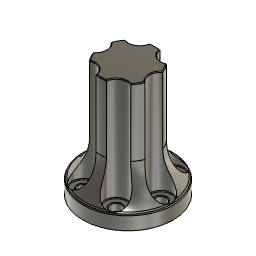
Motor_Shaft v4 (Autodesk Fusion 360 archive; units mm, degrees)
design "Motor_Shaft v4" references "Spring Washer BS 4464 - M4 - Type B Steel 100 HV Plain", "Forged Hexagon Socket Head Cap Screw ANSI B18.3.1M - M4x0.7 x 12 Steel Grade 8 Plain"
Autodesk Fusion 360 part; units mm, degrees
sketch "Sketch1" plane through (0, 0, 0) normal (0, 0, 1) x (1, 0, 0)
  circle A0 centre (0, 0) radius 16.5
  dimension "d1" = 33
  constraint coincident A0.centre origin
  measures "d1" diameter of A0
extrude "Extrude1" add sketch "Sketch1" along normal blind 5
sketch "Sketch2" plane through (0, 0, 5) normal (0, 0, 1) x (-1, 0, 0)
  circle A0 centre (0, 0) radius 16.5
  circle A1 centre (0, 0) radius 12 construction
  circle A2 centre (12, 0) radius 2.075
  circle A3 centre (6, 10.3923) radius 2.075
  circle A4 centre (-6, 10.3923) radius 2.075
  circle A5 centre (-12, 0) radius 2.075
  circle A6 centre (-6, -10.3923) radius 2.075
  circle A7 centre (6, -10.3923) radius 2.075
  circle A8 centre (0, 0) radius 10
  circle A9 centre (12, 0) radius 4.125
  circle A10 centre (6, 10.3923) radius 4.125
  circle A11 centre (-6, 10.3923) radius 4.125
  circle A12 centre (-12, 0) radius 4.125
  circle A13 centre (-6, -10.3923) radius 4.125
  circle A14 centre (6, -10.3923) radius 4.125
  dimension "d4" = 24
  dimension "d5" = 4.15
  dimension "d7" = 360
  dimension "d10" = 20
  dimension "d15" = 8.25
  dimension "d17" = 360
  constraint coincident A0.centre A1.centre
  constraint coincident A1 A2.centre
  constraint concentric A1 A8
  constraint concentric A2 A9
  measures "d4" diameter of A1
  measures "d5" diameter of A2
  measures "d10" diameter of A8
  measures "d15" diameter of A9
extrude "Extrude2" cut sketch "Sketch2" against normal blind 5.5 contours A2 A8 | A2 A8 | A3 A8 | A3 A8 | A7 A8 | A7 A8 | A4 A8 | A4 A8 | A6 A8 | A6 A8 | A5 A8 | A5 A8
extrude "Extrude3" add sketch "Sketch2" along normal blind 37 contours A2 A8 | A2 A8 A9 | A8 A9 A10 A11 A12 A13 A14 | A3 A8 A10 | A7 A8 A14 | A3 A8 | A7 A8 | A4 A8 A11 | A6 A8 A13 | A4 A8 | A6 A8 | A5 A8 A12 | A5 A8 picked at (9.9547, 0.1408) picked at (9.3357, 1.1161) picked at (3.7013, 8.643) picked at (3.7013, -8.643) picked at (4.987, 8.6378) picked at (4.987, -8.6378) picked at (-3.7013, 8.643) picked at (-3.7013, -8.643) picked at (-4.987, 8.6378) picked at (-4.987, -8.6378) picked at (-9.2988, 0.9985) picked at (-9.9741, 0)
sketch "Sketch3" plane through (0, 0, 0) normal (0, 1, 0) x (1, 0, 0)
  line L0 (-10, -5) -> (-16.5, -5)
  line L1 (-10, -5) -> (-10, -10)
  line L2 (-10, -10) -> (-16.5, -5)
  arc A0 (-10, -10) -> (-16.5, -5) centre (-15.1731, -10) ccw
  point P0 (-16.5, -5)
  point P1 (-9.9873, -5)
  point P2 (-9.9873, -5)
  dimension "d13" = 5
  constraint coincident P0 L0.end
  constraint perpendicular L0 L1
  constraint tangent L1 A0
  measures "d13" distance of L0.start L1.end
revolve "Revolve1" add sketch "Sketch3" angle 360 about axis through (0, 0, 1.75) along (0, 0, 1) contours L0 L1 A0 | L0 L2 A0
extrude "Extrude4" cut sketch "Sketch2" along normal blind 37 and the other way blind 1 contours A2 A8 | A2 A8 A9 | A2 A8 | A2 A8 A9 | A3 A8 A10 | A3 A8 A10 | A7 A8 A14 | A7 A8 A14 | A3 A8 | A3 A8 | A7 A8 | A7 A8 | A4 A8 A11 | A4 A8 A11 | A6 A8 A13 | A6 A8 A13 | A4 A8 | A4 A8 | A6 A8 | A6 A8 | A5 A8 A12 | A5 A8 A12 | A5 A8 | A5 A8
fillet "Fillet1" radius 15 6 edges at (0, -10, 10) (8.6603, -5, 10) (8.6603, 5, 10) (-8.6603, -5, 10) (-8.6603, 5, 10) (0, 10, 10)
sketch "Sketch4" plane through (0, 0, 0) normal (0, 0, -1) x (1, 0, 0)
  circle A0 centre (0, 0) radius 16.5
  circle A1 centre (0, 0) radius 15.25
  circle A2 centre (12, 0) radius 2.075
  circle A3 centre (-12, 0) radius 2.075
  circle A4 centre (6, 10.3923) radius 2.075
  circle A5 centre (6, -10.3923) radius 2.075
  circle A6 centre (-6, -10.3923) radius 2.075
  circle A7 centre (-6, 10.3923) radius 2.075
  dimension "d25" = 30.5
  constraint coincident A0.centre A1.centre
  measures "d25" diameter of A1
extrude "Extrude5" cut sketch "Sketch4" against normal blind 1 contours A1 | A2 | A3 | A4 | A5 | A6 | A7
chamfer "Chamfer1" distance 0.25 angle 45 1 faces at (-1.4005, 2.3241, 42)
chamfer "Chamfer1" distance 0.25 angle 45 6 faces at (3.9353, 10.5989, 3) (9.9353, 0.2066, 3) (-8.0647, 10.5989, 3) (-14.0647, 0.2066, 3) (3.9353, -10.1857, 3) (-8.0647, -10.1857, 3)
fillet "Fillet2" radius 0.25 1 edges at (-14.218, -5.5146, 1)
fillet "Fillet2" radius 0.5 1 edges at (-15.3834, -5.9667, 5)
fillet "Fillet2" radius 0.25 6 edges at (-2.1541, -11.884, 4) (9.8459, -11.884, 4) (-8.1541, -1.4917, 4) (-2.1541, 8.9006, 4) (9.8459, 8.9006, 4) (15.8459, -1.4917, 4)
thread "Thread1" [rolled back] thread offset 0 thread length 10
other "Washer7"
other "Washer8"
other "Washer9"
other "Washer10"
other "Washer11"
other "Washer12"
other "Screw13"
other "Screw14"
other "Screw15"
other "Screw16"
other "Screw17"
other "Screw18"

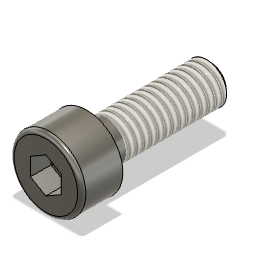
design "Forged Hexagon Socket Head Cap Screw ANSI B18.3.1M - M4x0.7 x 12 Steel Grade 8 Plain"
description: Forged Hexagon Socket Head Cap Screw ANSI B18.3.1M - M4x0.7 x 12
Autodesk Fusion 360 part; units mm, degrees
sketch "Sketch1" plane through (0, 0, 0) normal (0, 1, 0) x (1, 0, 0)
  line L0 (-2, 0) -> (-2, 12)
  line L1 (-2, 12) -> (0, 12)
  line L2 (0, 12) -> (0, -4)
  line L3 (-2, 0) -> (-3.5, 0)
  line L4 (-3.5, 0) -> (-3.5, -4)
  line L5 (-3.5, -4) -> (0, -4)
  dimension "d9" = 4
  dimension "d66" = 7
  dimension "d68" = 12
  dimension "d79" = 4
  constraint perpendicular L0 L1
  constraint collinear origin L1.end L2.end
  constraint perpendicular L0 L3
  constraint coincident origin L3
  constraint vertical L0
  constraint vertical L2
  constraint parallel L2 L4
  constraint coincident L2 L5.end
  constraint perpendicular L2 L5
  measures "d68" distance of origin L1.end
  measures "d79" distance of L3.end L4.end
revolve "Revolve1" add sketch "Sketch1" angle 360 about axis through (0, 0, -12) along (0, 0, 1)
ref_plane "WorkPlane1" through (0, 0, 4) normal (0, 0, 1) x (1, 0, 0)
sketch "Sketch6" plane through (0, 0, 4) normal (0, 0, 1) x (1, 0, 0)
  line L0 (-1.5, 0) -> (1.5, 0) construction
  line L1 (0, 0) -> (-1.5, 0.866)
  line L2 (-1.5, -0.866) -> (-1.5, 0.866)
  line L3 (-1.5, -0.866) -> (0, 0)
  dimension "d72" = 3
  dimension "d100" = 150
  constraint horizontal L0
  constraint midpoint L1.start L0
  constraint coincident L1.start L3.end
  constraint perpendicular L0 L2
  constraint midpoint L0.start L2
  constraint coincident L1.end L2.end
  measures "d72" distance of L0.start L0.end
  measures "d100" angle of L0 L1
extrude "Extrude1" cut sketch "Sketch6" against normal blind 2
pattern_circular "C-Pattern1" count 6 over 360 about axis through (0, 0, 1.75) along (0, 0, 1) of "Extrude1"
extrude "Extrude2" cut 1 faces at (0, -0.5774, 2) along direction (0, 0, -1) blind 2 draft -85
thread "Thread2" "ANSI Metric M Profile 4.0 M4x0.7 4g6g" major diameter 3.908 minor diameter 3.128 pitch 0.7 angle 60 resizes the face on face at (-1.9975, 0.0997, -8) from (0, 0, -1.8294) to (0, 0, -12)
fillet "Fillet4" radius 0.4 1 edges at (-3.2631, 1.2657, 4)
sketch "Sketch7" plane through (0, 0, 0) normal (0, 1, 0) x (1, 0, 0)
  line L0 (-2.04, 12) -> (-2.04, 11.5706)
  line L1 (-2.04, 11.5706) -> (-1.5706, 12)
  line L2 (0, 12) -> (0, -4)
  line L3 (-2.04, 12) -> (0, 12)
  dimension "d92" = 0.4294
  dimension "d98" = 1.5706
  dimension "d99" = 2.04
  constraint coincident L2.start L3.end
  constraint perpendicular L2 L3
  constraint coincident L1.end L3
  constraint perpendicular L0 L3
  measures "d92" vertical distance of L0.end L1.end
  measures "d98" horizontal distance of origin L1.end
  measures "d99" distance of origin L0
revolve "Revolve3" cut sketch "Sketch7" angle 360 about axis through (0, 0, 1.75) along (0, 0, 1)
equation "d9 = adsk_nomdia"
equation "adsk_nomlen = 12.00 mm"
equation "adsk_headh = 4.00 mm"
equation "adsk_headdia = 7.00 mm"
equation "adsk_nomdia = 4.00 mm"
equation "adsk_philwidth = 3.00 mm"
equation "d31 = -adsk_phildepth"
equation "adsk_phildepth = 2.00 mm"
equation "d66 = adsk_headdia"
equation "d68 = adsk_nomlen"
equation "d71 = adsk_headh"
equation "d72 = adsk_philwidth"
equation "d76 = -adsk_phildepth"
equation "d79 = adsk_headh"
equation "adsk_thrlen = 10.170585 mm"
equation "d84 = adsk_thrlen"
equation "d86 = adsk_nomdia * 0.1"
equation "d92 = adsk_startlen"
equation "adsk_startlen = 0.429415 mm"
equation "adsk_endpointdia = 3.14117 mm"
equation "d98 = adsk_endpointdia / 2"
equation "d99 = adsk_nomdia * 0.51"

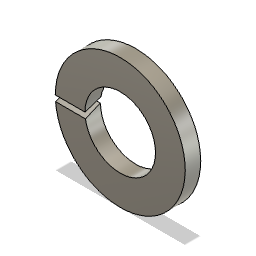
design "Spring Washer BS 4464 - M4 - Type B Steel 100 HV Plain"
description: Spring Washer BS 4464 - M4 - Type B
Autodesk Fusion 360 part; units mm, degrees
sketch "Sketch1" plane through (0, 0, 0) normal (0, 0, 1) x (1, 0, 0)
  circle A0 centre (0, 0) radius 3.775
  circle A1 centre (0, 0) radius 2.05
  dimension "d4" = 7.55
  dimension "d5" = 4.1
  constraint coincident A0.centre A1.centre
  measures "d4" diameter of A0
  measures "d5" diameter of A1
extrude "Extrude1" add sketch "Sketch1" along normal blind 0.9
ref_plane "WorkPlane1" through (12.125, 0, 0) normal (0, -0.34202, 0.939693) x (1, 0, 0)
ref_plane "WorkPlane2" through (12.125, -0.1539, 0.4229) normal (0, -0.34202, 0.939693) x (1, 0, 0)
sketch "Sketch2" plane through (12.125, -0.1539, 0.4229) normal (0, -0.34202, 0.939693) x (1, 0, 0)
  ellipse E0 centre (-12.125, 0.3078) end of major axis (-8.35, 0.3078) minor radius 3.5473
  ellipse E1 centre (-12.125, 0) end of major axis (-8.35, 0) minor radius 3.5473
  line L0 (-12.125, 0.3078) -> (-12.125, 0)
  line L1 (-12.125, 0.3078) -> (-16.051, 0.3078)
  line L2 (-12.125, 0) -> (-16.051, 0)
  line L3 (-16.051, 0) -> (-16.051, 0.3078)
  dimension "d15" = 3.926
  constraint coincident E0.centre L0.start
  constraint coincident E1.centre L0.end
  constraint perpendicular L0 L1
  constraint perpendicular L0 L2
  constraint vertical L3
  measures "d15" distance of L0 L3
extrude "Extrude2" cut sketch "Sketch2" along normal through all and the other way through all contours E0 E1 L1 | E0 E1 L1 L2 L3 | E0 E1 L0 L1 L2 | E0 E1 L2 picked at (-15.8916, 0.295) picked at (-13.3786, 0.1026) picked at (-15.8916, 0.0128)
equation "adsk_woutdia = 7.55 mm"
equation "adsk_windia = 4.10 mm"
equation "adsk_wthick = 0.90 mm"
equation "d4 = adsk_woutdia"
equation "d5 = adsk_windia"
equation "d6 = adsk_wthick"
equation "d13 = adsk_wthick / 2"
equation "d15 = adsk_woutdia * 0.52"
equation "d34 = adsk_wthick"
